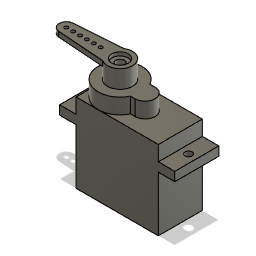
9g Servo' v2 (Autodesk Fusion 360 design; units mm, degrees)
Autodesk Fusion 360 part; units mm, degrees
note: some values were not read from the file. Set by a fixed rule: which sketch regions a step uses.
sketch "Sketch1" plane through (0, 0, 0) normal (0, 1, 0) x (1, 0, 0)
  line L0 (-20, 10) -> (3, 10)
  line L1 (3, 10) -> (3, -2.3)
  line L2 (3, -2.3) -> (-20, -2.3)
  line L3 (-20, -2.3) -> (-20, 10)
  dimension "d1" = 23
  dimension "d2" = 12.3
  constraint horizontal L0
  constraint vertical L1
  constraint horizontal L2
  constraint vertical L3
  measures "d1" distance of L0.start L0.end
  measures "d2" distance of L0.start L2.end
extrude "Extrude1" add sketch "Sketch1" along normal blind 15.4 makes body 1
sketch "Sketch2" plane through (0, 15.4, 0) normal (0, 1, 0) x (-1, 0, 0)
  line L0 (20, 2.3) -> (-3, 2.3)
  line L1 (-3, 2.3) -> (-3, -10)
  line L2 (-3, -10) -> (20, -10)
  line L3 (20, -10) -> (20, 2.3)
  line L4 (24.6, -10) -> (-7.6, -10)
  line L5 (-7.6, -10) -> (-7.6, 2.3)
  line L6 (-7.6, 2.3) -> (24.6, 2.3)
  line L7 (24.6, 2.3) -> (24.6, -10)
  line L8 (24.6, -10) -> (-7.6, 2.3) construction
  line L9 (-7.6, -10) -> (24.6, 2.3) construction
  line L10 (20, -3.85) -> (24.6, -3.85) construction
  line L11 (-3, -3.85) -> (-7.6, -3.85) construction
  circle A0 centre (-5.3, -3.85) radius 1
  circle A1 centre (22.3, -3.85) radius 1
  point P0 (8.5, -3.85)
  dimension "d5" = 32.2
  dimension "d6" = 2
  dimension "d7" = 2
  constraint horizontal L4
  constraint perpendicular L4 L5
  constraint parallel L4 L6
  constraint parallel L5 L7
  constraint coincident L8 P0
  constraint coincident L9 P0
  constraint midpoint L3 L10.start
  constraint midpoint L7 L10.end
  constraint midpoint L1 L11.start
  constraint midpoint L5 L11.end
  constraint midpoint L11 A0.centre
  constraint midpoint L10 A1.centre
  measures "d5" distance of L5.end L6.end
  measures "d6" diameter of A0
  measures "d7" diameter of A1
extrude "Extrude2" add sketch "Sketch2" along normal blind 2.5 bodies 1
sketch "Sketch3" plane through (0, 17.9, 0) normal (0, 1, 0) x (-1, 0, 0)
  circle A0 centre (-5.3, -3.85) radius 1
  circle A1 centre (22.3, -3.85) radius 1
  line L0 (24.6, 2.3) -> (-7.6, 2.3)
  line L1 (-7.6, 2.3) -> (-7.6, -10)
  line L2 (-7.6, -10) -> (24.6, -10)
  line L3 (24.6, -10) -> (24.6, 2.3)
  line L4 (-3, 2.3) -> (20, 2.3)
  line L5 (20, 2.3) -> (20, -10)
  line L6 (20, -10) -> (-3, -10)
  line L7 (-3, -10) -> (-3, 2.3)
extrude "Extrude3" add sketch "Sketch3" along normal blind 4.2 contours L0 L2 L4 L5 L6 L7 bodies 1
sketch "Sketch4" plane through (0, 22.1, 0) normal (0, 1, 0) x (-1, 0, 0)
  line L0 (-3, -10) -> (20, -10)
  line L1 (20, -10) -> (20, 2.3)
  line L2 (20, 2.3) -> (-3, 2.3)
  line L3 (-3, 2.3) -> (-3, -10)
  circle A0 centre (13.85, -3.85) radius 6.15
  circle A1 centre (7, -4) radius 2.8
  line L4 (12.5, -6.8) -> (1.5, -6.8)
  line L5 (1.5, -6.8) -> (1.5, -1.2)
  line L6 (1.5, -1.2) -> (12.5, -1.2)
  line L7 (12.5, -1.2) -> (12.5, -6.8)
  line L8 (12.5, -6.8) -> (1.5, -1.2) construction
  line L9 (1.5, -6.8) -> (12.5, -1.2) construction
  point P0 (7, -4)
  dimension "d12" = 5.6
  dimension "d13" = 5.6
  constraint tangent L0 A0
  constraint tangent L2 A0
  constraint tangent L1 A0
  constraint horizontal L4
  constraint perpendicular L4 L5
  constraint parallel L4 L6
  constraint parallel L5 L7
  constraint coincident L8 P0
  constraint coincident L9 P0
  constraint coincident P0 A1.centre
  measures "d12" diameter of A1
  measures "d13" distance of L4.end L5.end
extrude "Extrude4" add sketch "Sketch4" along normal blind 4.3 contours A0 L4 L6 L7 | A0 A1 L4 | A0 A1 L4 L6 L7 | A0 A1 | A0 A1 | A0 A1 L6 bodies 1
sketch "Sketch5" plane through (0, 26.4, 0) normal (0, 1, 0) x (-1, 0, 0)
  arc A0 (7, -1.2) -> (7, -6.8) centre (7, -4) ccw
  line L0 (7, -6.8) -> (8.4537, -6.8)
  arc A1 (8.4537, -6.8) -> (8.3002, -1.2) centre (13.85, -3.85) ccw
  line L1 (8.3002, -1.2) -> (7, -1.2)
  circle A2 centre (13.85, -3.85) radius 3.5
  dimension "d16" = 7
  constraint concentric A1 A2
  measures "d16" diameter of A2
extrude "Extrude5" add sketch "Sketch5" along normal blind 5 contours A2 bodies 1
sketch "Sketch6" plane through (0, 31.4, 0) normal (0, 1, 0) x (-1, 0, 0)
  circle A0 centre (13.85, -3.85) radius 3.5
  line L0 (13.85, -3.85) -> (28.85, -3.85)
  circle A1 centre (28.85, -3.85) radius 2
  line L1 (15.7335, -6.8) -> (15.7335, -0.9)
  line L2 (15.7335, -6.8) -> (28.9937, -5.8448)
  line L3 (15.7335, -0.9) -> (28.9937, -1.8552)
  dimension "d19" = 15
  dimension "d20" = 4
  dimension "d21" = 5.9
  constraint coincident A0.centre L0.start
  constraint horizontal L0
  constraint coincident L0.end A1.centre
  constraint vertical L1
  constraint coincident A0 L1.start
  constraint coincident A0 L1.end
  constraint coincident A1 L2.end
  constraint tangent A1 L2
  constraint coincident A1 L3.end
  constraint tangent A1 L3
  measures "d19" distance of A0.centre L0.end
  measures "d20" diameter of A1
  measures "d21" distance of L1.start L1.end
extrude "Extrude6" add sketch "Sketch6" against normal blind 1.4 contours A0 L0 A1 L2 | A0 L0 A1 L3 | A1 bodies 1
sketch "Sketch7" plane through (0, 31.4, 0) normal (0, 1, 0) x (-1, 0, 0)
  arc A0 (15.7335, -0.9) -> (15.7335, -6.8) centre (13.85, -3.85) ccw
  line L0 (15.7335, -6.8) -> (28.9937, -5.8448)
  arc A1 (28.9937, -5.8448) -> (28.9937, -1.8552) centre (28.85, -3.85) ccw
  line L1 (28.9937, -1.8552) -> (15.7335, -0.9)
  circle A2 centre (13.85, -3.85) radius 3.5 construction
  circle A3 centre (28.85, -3.85) radius 0.5
  line L2 (17.35, -3.85) -> (28.85, -3.85) construction
  circle A4 centre (26.9333, -3.85) radius 0.5
  circle A5 centre (25.0167, -3.85) radius 0.5
  circle A6 centre (23.1, -3.85) radius 0.5
  circle A7 centre (21.1833, -3.85) radius 0.5
  circle A8 centre (19.2667, -3.85) radius 0.5
  circle A9 centre (17.35, -3.85) radius 0.5
  dimension "d24" = 1
  dimension "d27" = -11.5
  dimension "d28" = 0
  constraint concentric A0 A2
  constraint coincident A0.start A2
  constraint concentric A1 A3
  constraint coincident A2 L2.start
  constraint coincident A1.centre A3.centre
  constraint horizontal L2
  measures "d24" diameter of A3
extrude "Extrude7" cut sketch "Sketch7" against normal up to surface (1.4 mm away) contours A3 | A4 | A5 | A6 | A7 | A8 bodies 1
sketch "Sketch8" plane through (0, 31.4, 0) normal (0, 1, 0) x (-1, 0, 0)
  circle A0 centre (25.0167, -3.85) radius 0.5
  circle A1 centre (19.2667, -3.85) radius 0.5
  circle A2 centre (26.9333, -3.85) radius 0.5
  circle A3 centre (23.1, -3.85) radius 0.5
  circle A4 centre (21.1833, -3.85) radius 0.5
  circle A5 centre (28.85, -3.85) radius 0.5
  arc A6 (15.7335, -0.9) -> (15.7335, -6.8) centre (13.85, -3.85) ccw
  line L0 (15.7335, -6.8) -> (28.9937, -5.8448)
  arc A7 (28.9937, -5.8448) -> (28.9937, -1.8552) centre (28.85, -3.85) ccw
  line L1 (28.9937, -1.8552) -> (15.7335, -0.9)
  circle A8 centre (13.85, -3.85) radius 2.3
  dimension "d31" = 4.6
  constraint concentric A6 A8
  measures "d31" diameter of A8
extrude "Extrude8" cut sketch "Sketch8" against normal blind 1 contours A8 bodies 1
sketch "Sketch9" plane through (0, 30.4, 0) normal (0, 1, 0) x (-1, 0, 0)
  circle A0 centre (13.85, -3.85) radius 2.3
  circle A1 centre (13.85, -3.85) radius 1.2
  dimension "d34" = 2.4
  constraint concentric A0 A1
  measures "d34" diameter of A1
extrude "Extrude9" cut sketch "Sketch9" against normal blind 3 contours A1 bodies 1
copy_body "Body->Comp1" bodies 1 removing the originals makes body 2 in component "Servo"
component "Servo" placed x (1, 0, 0) y (0, 1, 0) z (0, 0, 1) at (0, 0, 0)
